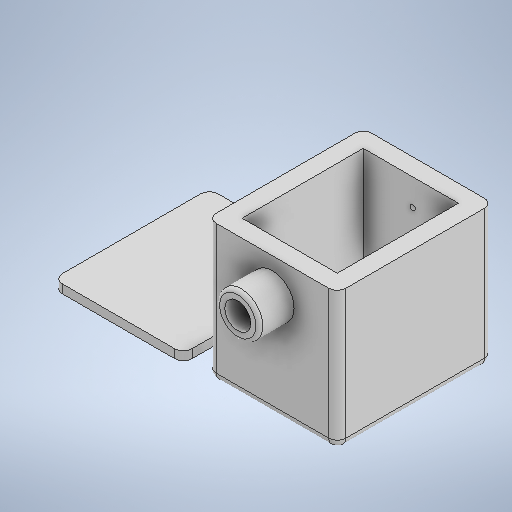
# Autodesk Inventor part: Alcoholimetro
Saved by Autodesk Inventor 2025.4 (Build 294407000, 407)
## iProperties
Created: 2026-05-31
Part Number: Alcoholimetro
Material: Genérico
Document SubType Name: Modeling
Designer: Leo Pacheco
Density: 1 g/cm^3
Appearance: Valor por defecto
Author: Leo Pacheco
## iProperties of the stored document Alcoholimetro_3DPrint.ipt
Created: 2026-05-31
Part Number: Alcoholimetro_3DPrint
Material: Genérico
Document SubType Name: Modeling
Designer: Leo Pacheco
Density: 1 g/cm^3
Appearance: Valor por defecto
Author: Leo Pacheco
Autodesk Inventor part; units mm, degrees
ref_plane "YZ Plane" through (0, 0, 0) normal (1, 0, 0) x (0, 1, 0)
ref_plane "XZ Plane" through (0, 0, 0) normal (0, 1, 0) x (-1, 0, 0)
ref_plane "XY Plane" through (0, 0, 0) normal (0, 0, 1) x (1, 0, 0)
sketch "Boceto1" plane through (0, 0, 0) normal (0, 1, 0) x (-1, 0, 0)
  line L0 (0, 0) -> (75, 0)
  line L1 (75, 0) -> (75, -90)
  line L2 (75, -90) -> (0, -90)
  line L3 (0, -90) -> (0, 0)
  dimension "d0" = 75
  dimension "d1" = 90
  constraints: 8 end point, 2 parallel, 1 horizontal, 1 perpendicular
  measures "d0" distance of L1.end L2.end
  measures "d1" distance of L0.end L1.end
extrude "Extrusión1" add sketch "Boceto1" along normal blind 10
sketch "Boceto2" plane through (0, 10, 0) normal (0, 1, 0) x (1, 0, 0)
  line L0 (-10, 10) -> (-65, 10)
  line L1 (-65, 10) -> (-65, 80)
  line L2 (-65, 80) -> (-10, 80)
  line L3 (-10, 80) -> (-10, 10)
  line L4 (-75, 0) -> (0, 0) projected
  line L5 (0, 90) -> (-75, 90) projected
  line L6 (0, 0) -> (0, 90) projected
  line L7 (-75, 90) -> (-75, 0) projected
  line L8 (0, 0) -> (-75, 0)
  line L9 (-75, 0) -> (-75, 90)
  line L10 (-75, 90) -> (0, 90)
  line L11 (0, 90) -> (0, 0)
  dimension "d4" = 10
  dimension "d5" = 10
  dimension "d6" = 10
  dimension "d7" = 10
  constraints: 16 end point, 4 parallel, 2 horizontal, 2 perpendicular
  measures "d4" distance between parallel lines of L4 L0
  measures "d5" distance between parallel lines of L5 L2
  measures "d6" distance between parallel lines of L6 L3
  measures "d7" distance between parallel lines of L7 L1
extrude "Extrusión2" add sketch "Boceto2" along normal blind 70
sketch "Boceto3" plane through (0, 0, -90) normal (0, 0, -1) x (-1, 0, 0)
  line L0 (0, 0) -> (0, 80) projected
  line L1 (0, 10) -> (80.4696, 10)
  line L2 (0, 0) -> (75, 0) projected
  line L3 (65, 10) -> (65, 80) projected
  line L4 (65, 80) -> (65, 10)
  line L5 (10, 10) -> (10, 80) projected
  line L6 (10, 80) -> (10, 10)
  line L7 (21.6, 10) -> (33.6, 10)
  line L8 (33.6, 10) -> (33.6, 22)
  line L9 (33.6, 22) -> (21.6, 22)
  line L10 (21.6, 22) -> (21.6, 10)
  line L11 (51.6, 10) -> (61, 10)
  line L12 (61, 10) -> (61, 19.4)
  line L13 (61, 19.4) -> (51.6, 19.4)
  line L14 (51.6, 19.4) -> (51.6, 10)
  dimension "d10" = 10
  dimension "d11" = 12
  dimension "d12" = 9.4
  dimension "d13" = 18
  dimension "d14" = 4
  constraints: 22 end point, 5 equal length, 5 perpendicular, 3 horizontal, 3 point on line
  measures "d10" distance between parallel lines of L2 L1
  measures "d11" distance of L8.end L9.end
  measures "d12" distance of L12.end L13.end
  measures "d13" distance between parallel lines of L8 L14
  measures "d14" distance between parallel lines of L3 L12
extrude "Extrusión3" cut sketch "Boceto3" against normal blind 70
sketch "Boceto4" plane through (-75, 0, 0) normal (0, 0, 1) x (1, 0, 0)
  point P0 (75, 0)
  point P1 (38.6263, 64.6608)
hole "Agujero1" at (-36.3737, 64.6608, 0) direction (0, 0, -1) diameter 3 end through all
sketch "Boceto5" plane through (-75, 0, 0) normal (0, 0, 1) x (1, 0, 0)
  circle A0 centre (37.5, 60) radius 7.5
  line L0 (0, 80) -> (75, 80) projected
  point P0 (75, 0)
  point P1 (37.5, 80)
  dimension "d24" = 20
  dimension "d25" = 15
  constraints: 1 centre point, 1 midpoint, 1 vertical alignment
  measures "d24" distance from line of L0 A0.centre
  measures "d25" diameter of A0
extrude "Extrusión4" cut sketch "Boceto5" against normal blind 15
sketch "Boceto6" plane through (-75, 0, 0) normal (0, 0, 1) x (1, 0, 0)
  circle A0 centre (37.5, 60) radius 7.5 projected
  circle A1 centre (37.5, 60) radius 12.5
  circle A2 centre (37.5, 60) radius 7.5
  point P0 (75, 0)
  dimension "d28" = 5
  constraints: 2 centre point, 2 coincident, 1 concentric
  measures "d28" radial gap between concentric circles of A1 A0
extrude "Extrusión5" add sketch "Boceto6" along normal blind 20
fillet "Empalme1" radius 2 1 edges at (-50, 60, 20)
fillet "Empalme2" radius 5 8 edges at (0, 0, -45) (0, 40, 0) (-75, 40, 0) (-37.5, 0, 0) (0, 40, -90) (-75, 40, -90) (-37.5, 0, -90) (-75, 0, -45)
sketch "Boceto7" plane through (0, 0, 0) normal (0, 1, 0) x (-1, 0, 0)
  line L0 (94.2127, -0.2655) -> (159.2127, -0.2655)
  line L1 (164.2127, -5.2655) -> (164.2127, -85.2655)
  line L2 (159.2127, -90.2655) -> (94.2127, -90.2655)
  line L3 (89.2127, -85.2655) -> (89.2127, -5.2655)
  line L4 (0, -5) -> (0, -85) projected
  line L5 (75, -85) -> (75, -5) projected
  arc A0 (94.2127, -0.2655) -> (89.2127, -5.2655) centre (94.2127, -5.2655) ccw
  arc A1 (164.2127, -5.2655) -> (159.2127, -0.2655) centre (159.2127, -5.2655) ccw
  arc A2 (159.2127, -90.2655) -> (164.2127, -85.2655) centre (159.2127, -85.2655) ccw
  arc A3 (89.2127, -85.2655) -> (94.2127, -90.2655) centre (94.2127, -85.2655) ccw
  point P0 (0, 0)
  point P1 (89.2127, -45.2655)
  dimension "d33" = 75
  dimension "d34" = 75
  dimension "d35" = 90
  dimension "d36" = 5
  constraints: 8 end point, 8 point on circle, 8 tangent, 4 centre point, 3 equal radius, 2 parallel, 1 horizontal, 1 midpoint, 1 perpendicular
  measures "d33" distance between parallel lines of L4 L5
  measures "d34" distance from line of L1 point (89.213, -45.266)
  measures "d35" distance between parallel lines of L2 L0
  measures "d36" radius of A0
extrude "Extrusión6" add sketch "Boceto7" along normal blind 5
